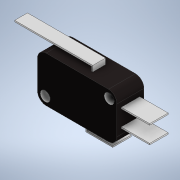
# Autodesk Inventor part: switch_V_152_1A5_KM
Saved by Autodesk Inventor 2022 (Build 260153070, 153G)
## iProperties
Created: 2022-04-01
Part Number: switch_V_152_1A5_KM
Material: 一般
Document SubType Name: Modeling
Designer: zegi
Density: 1 g/cm^3
Appearance: 既定
Author: zegi
Autodesk Inventor part; units mm, degrees
ref_plane "YZ Plane" through (0, 0, 0) normal (1, 0, 0) x (0, 1, 0)
ref_plane "XZ Plane" through (0, 0, 0) normal (0, 1, 0) x (-1, 0, 0)
ref_plane "XY Plane" through (0, 0, 0) normal (0, 0, 1) x (1, 0, 0)
sketch "スケッチ1" plane through (0, 0, 0) normal (0, 0, 1) x (1, 0, 0)
  line L0 (0, 0) -> (28, 0)
  line L1 (28, 0) -> (28, 16)
  line L2 (28, 16) -> (0, 16)
  line L3 (0, 16) -> (0, 0)
  line L4 (0, 11.25) -> (0, 4.75)
  dimension "d0" = 28
  dimension "d1" = 16
  dimension "d2" = 6.5
  dimension "d3" = 4.75
  constraints: 10 end point, 2 parallel, 2 point on line, 1 horizontal, 1 perpendicular
  measures "d0" distance of L2.end L1.end
  measures "d1" distance of L1.end L0.end
  measures "d2" distance of L4.start L4.end
  measures "d3" distance of L2.end L4.start
extrude "押し出し1" add sketch "スケッチ1" along normal blind 9.5
sketch "スケッチ2" plane through (28, 0, 0) normal (1, 0, 0) x (0, 0, -1)
  line L0 (0, 16) -> (0, 0) projected
  line L1 (0, 11.25) -> (0, 4.75)
  line L2 (0, 16) -> (-9.5, 16) projected
  line L3 (-8, 16) -> (-1.5, 16)
  line L4 (-8, 11.25) -> (-1.5, 11.25)
  line L5 (-1.5, 11.25) -> (-1.5, 10.75)
  line L6 (-1.5, 10.75) -> (-8, 10.75)
  line L7 (-8, 10.75) -> (-8, 11.25)
  line L8 (-8, 4.75) -> (-1.5, 4.75)
  line L9 (-1.5, 4.75) -> (-1.5, 5.25)
  line L10 (-1.5, 5.25) -> (-8, 5.25)
  line L11 (-8, 5.25) -> (-8, 4.75)
  dimension "d6" = 6.5
  dimension "d7" = 4.75
  dimension "d8" = 6.5
  dimension "d9" = 1.5
  dimension "d10" = 0.5
  dimension "d11" = 0.5
  constraints: 20 end point, 6 point on line, 4 parallel, 2 horizontal, 2 perpendicular
  measures "d6" distance of L1.start L1.end
  measures "d7" distance of L0.start L1.start
  measures "d8" distance of L3.start L3.end
  measures "d9" distance of L2.end L3.start
  measures "d10" distance of L4.end L5.end
  measures "d11" distance of L9.end L8.end
extrude "押し出し2" add sketch "スケッチ2" along normal blind 10
sketch "スケッチ3" plane through (0, 16, 0) normal (0, 1, 0) x (1, 0, 0)
  line L0 (0, -9.5) -> (28, -9.5) projected
  line L1 (17, -9.5) -> (17, 0)
  line L2 (28, 0) -> (28, -9.5) projected
  line L3 (17, -7) -> (17, -2.5)
  line L4 (17, -7) -> (16.5, -7)
  line L5 (16.5, -7) -> (16.5, -2.5)
  line L6 (16.5, -2.5) -> (17, -2.5)
  line L7 (17, -2.5) -> (17, -7)
  point P0 (0, 0)
  dimension "d14" = 11
  dimension "d15" = 4.5
  dimension "d16" = 2.5
  dimension "d17" = 0.5
  constraints: 12 end point, 3 point on line, 2 parallel, 1 horizontal, 1 perpendicular, 1 vertical
  measures "d14" distance between parallel lines of L2 L1
  measures "d15" distance of L3.start L3.end
  measures "d16" distance from line of L0 L3.start
  measures "d17" distance of L5.end L6.end
extrude "押し出し3" add sketch "スケッチ3" along normal blind 2
sketch "スケッチ4" plane through (16.5, 16, 2.5) normal (-1, 0, 0) x (0, 0, 1)
  line L0 (0, 2) -> (4.5, 2) projected
  line L1 (4.5, 0) -> (4.5, 2) projected
  line L2 (0, 2) -> (4.5, 2)
  line L3 (4.5, 2) -> (4.5, 1.5)
  line L4 (4.5, 1.5) -> (0, 1.5)
  line L5 (0, 1.5) -> (0, 2)
  point P0 (-2.5, -16)
  dimension "d20" = 0.5
  constraints: 8 end point, 2 parallel, 1 horizontal, 1 perpendicular, 1 point on line
  measures "d20" distance of L2.end L3.end
extrude "押し出し4" add sketch "スケッチ4" along normal blind 27
sketch "スケッチ5" plane through (0, 0, 0) normal (0, -1, 0) x (1, 0, 0)
  line L0 (28, 9.5) -> (0, 9.5) projected
  line L1 (28, 0) -> (0, 0) projected
  line L2 (15.5, 9.5) -> (15.5, 0)
  line L3 (0, 0) -> (0, 9.5) projected
  line L4 (15.5, 8) -> (15.5, 1.5)
  line L5 (15.5, 8) -> (16, 8)
  line L6 (16, 8) -> (16, 1.5)
  line L7 (16, 1.5) -> (15.5, 1.5)
  line L8 (15.5, 1.5) -> (15.5, 8)
  dimension "d23" = 15.5
  dimension "d24" = 6.5
  dimension "d25" = 1.5
  dimension "d26" = 0.5
  constraints: 12 end point, 4 point on line, 2 parallel, 2 perpendicular, 1 horizontal
  measures "d23" distance between parallel lines of L3 L2
  measures "d24" distance of L4.start L4.end
  measures "d25" distance from line of L0 L4.start
  measures "d26" distance of L6.end L7.end
extrude "押し出し5" add sketch "スケッチ5" along normal blind 2.5 contours L5 L6 L7 L2
sketch "スケッチ6" plane through (16, 0, 8) normal (1, 0, 0) x (0, 0, -1)
  line L0 (0, -2.5) -> (6.5, -2.5) projected
  line L1 (0, 0) -> (0, -2.5) projected
  line L2 (6.5, -2.5) -> (0, -2.5)
  line L3 (0, -2.5) -> (0, -2)
  line L4 (0, -2) -> (6.5, -2)
  line L5 (6.5, -2) -> (6.5, -2.5)
  point P0 (8, 0)
  dimension "d29" = 0.5
  constraints: 8 end point, 2 parallel, 1 horizontal, 1 perpendicular, 1 point on line
  measures "d29" distance of L2.end L3.end
extrude "押し出し6" add sketch "スケッチ6" along normal blind 9
sketch "スケッチ7" plane through (0, 0, 0) normal (0, 0, -1) x (-1, 0, 0)
  line L0 (0, 16) -> (0, 0) projected
  line L1 (-28, 16) -> (0, 16) projected
  line L2 (-28, 0) -> (-28, 16) projected
  line L3 (0, 0) -> (-28, 0) projected
  point P0 (-2.75, 2.75)
  point P1 (-25.25, 13.25)
  dimension "d32" = 2.75
  dimension "d34" = 2.75
  dimension "d35" = 13.25
  dimension "d43" = 2.75
  measures "d32" distance from line of L0 point (-2.75, 2.75)
  measures "d34" distance from line of L2 point (-25.25, 13.25)
  measures "d35" distance from line of L3 point (-25.25, 13.25)
  measures "d43" distance from line of L3 point (-2.75, 2.75)
hole "穴1" at (2.75, 2.75, 0) at (25.25, 13.25, 0) direction (0, 0, 1) diameter 3.5 end through all
fillet "フィレット1" radius 3 4 edges at (0, 0, 4.75) (0, 16, 4.75) (28, 16, 4.75) (28, 0, 4.75)
equation "\"d34\" = d32"
equation "\"d43\" = d32"
equation "\"d33\" = d32"
